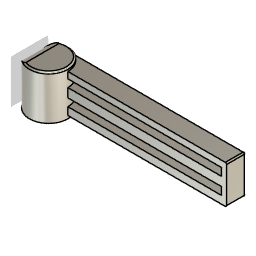
Link1 v24 (Autodesk Fusion 360 design; units mm, degrees)
Autodesk Fusion 360 part; units mm, degrees
sketch "Boceto1" plane through (0, 0, 0) normal (0, 1, 0) x (1, 0, 0)
  circle A0 centre (0, 0) radius 75.5
  dimension "d1" = 151
  constraint coincident A0.centre origin
  measures "d1" diameter of A0
extrude "Extruir1" add sketch "Boceto1" along normal blind 214.5
sketch "Boceto2" plane through (0, 0, 0) normal (1, 0, 0) x (0, 0, -1)
  line L0 (0, 201.5) -> (75, 201.5)
  line L1 (75, 201.5) -> (75, 51.5)
  line L2 (75, 51.5) -> (0, 51.5)
  line L3 (0, 51.5) -> (0, 201.5)
  line L4 (0, 176.5) -> (30, 176.5)
  line L5 (30, 176.5) -> (30, 146.5)
  line L6 (30, 146.5) -> (0, 146.5)
  line L7 (0, 146.5) -> (0, 176.5)
  line L8 (0, 111.5) -> (30, 111.5)
  line L9 (30, 111.5) -> (30, 81.5)
  line L10 (30, 81.5) -> (0, 81.5)
  line L11 (0, 81.5) -> (0, 111.5)
  point P0 (0, 214.5)
  dimension "d11" = 75
  dimension "d12" = 150
  dimension "d13" = 30
  dimension "d14" = 30
  dimension "d15" = 25
  dimension "d16" = 30
  dimension "d19" = 38
  dimension "d20" = 35
  constraint horizontal L0
  constraint vertical L1
  constraint horizontal L2
  constraint vertical L3
  constraint horizontal L4
  constraint vertical L5
  constraint horizontal L6
  constraint vertical L7
  constraint coincident L3 L4.start
  constraint horizontal L8
  constraint vertical L9
  constraint horizontal L10
  constraint vertical L11
  constraint coincident L3 L8.start
  measures "d11" distance of L0.start L0.end
  measures "d12" distance of L0.start L2.end
  measures "d13" distance of L4.start L4.end
  measures "d14" distance of L4.start L6.end
  measures "d15" distance of L0 L4
  measures "d16" distance of L2 L10
  measures "d19" distance of L4.start P0
  measures "d20" distance of L6 L8
sketch "Boceto3" plane through (0, 0, 0) normal (0, 0, 1) x (1, 0, 0)
sketch "Boceto4" plane through (0, 0, 0) normal (0, 0, 1) x (1, 0, 0)
  line L0 (-80, 0) -> (-80, 40)
  line L1 (-80, 40) -> (90, 40)
  line L2 (90, 40) -> (90, 0)
  line L3 (90, 0) -> (-80, 0)
  dimension "d8" = 40
  constraint vertical L0
  constraint perpendicular L0 L1
  constraint perpendicular L1 L2
  constraint perpendicular L0 L3
  measures "d8" distance of L0.start L0.end
extrude "Extruir3" cut sketch "Boceto4" along normal through all and the other way through all
extrude "Extruir4" add sketch "Boceto2" along normal blind 700 contours L0 L1 L2 L3 L4 L5 L6 L8 L9 L10
sketch "Boceto5" plane through (700, 0, 0) normal (1, 0, 0) x (0, 0, -1)
  line L0 (0, 111.5) -> (30, 111.5)
  line L1 (30, 111.5) -> (30, 81.5)
  line L2 (30, 81.5) -> (0, 81.5)
  line L3 (0, 81.5) -> (0, 51.5)
  line L4 (0, 51.5) -> (75, 51.5)
  line L5 (75, 51.5) -> (75, 201.5)
  line L6 (75, 201.5) -> (0, 201.5)
  line L7 (0, 201.5) -> (0, 176.5)
  line L8 (0, 176.5) -> (30, 176.5)
  line L9 (30, 176.5) -> (30, 146.5)
  line L10 (30, 146.5) -> (0, 146.5)
  line L11 (0, 146.5) -> (0, 111.5)
  line L12 (0, 176.5) -> (30, 176.5)
  line L13 (30, 176.5) -> (30, 146.5)
  line L14 (30, 146.5) -> (0, 146.5)
  line L15 (0, 146.5) -> (0, 176.5)
  line L16 (0, 111.5) -> (30, 111.5)
  line L17 (30, 111.5) -> (30, 81.5)
  line L18 (30, 81.5) -> (0, 81.5)
  line L19 (0, 81.5) -> (0, 111.5)
  constraint horizontal L12
  constraint vertical L13
  constraint horizontal L14
  constraint vertical L15
  constraint coincident L9.end L10.start
  constraint coincident L7.end L8.start
  constraint horizontal L16
  constraint vertical L17
  constraint horizontal L18
  constraint vertical L19
  constraint coincident L1.end L2.start
  constraint coincident L0.start L11.end
extrude "Extruir5" add sketch "Boceto5" against normal blind 20 contours L0 L1 L2 L16 L17 L18 L19 | L8 L9 L10 L12 L13 L14 L15
fillet "Empalme1" radius 6 1 edges at (-70.3907, 214.5, 27.302)
fillet "Empalme2" radius 5 1 edges at (700, 126.5, -75)
sketch "Boceto6" plane through (0, 0, 0) normal (0, 0, 1) x (1, 0, 0)
  spline S0 degree 5 poles (-140, 52.837) (-135.0375, 50.832) (-125.6476, 47.773) (-113.1693, 46.0387) (-99.7627, 49.465) (-88.3105, 63.072) (-81.5845, 84.6239) (-78.372, 111.348) (-76.0143, 137.2593) (-73.0835, 159.3989) (-68.896, 176.8089) (-63.175, 189.8686) (-55.7119, 199.6225) (-45.9985, 207.1017) (-32.9917, 212.8204) (-15.4222, 216.979) (3.2966, 219.0404) (20.4042, 219.8255) (33.2311, 220) (40, 220) knots 0 0 0 0 0 0 0.066667 0.133333 0.2 0.266667 0.333333 0.4 0.466667 0.533333 0.6 0.666667 0.733333 0.8 0.866667 0.933333 1 1 1 1 1 1
  line L0 (-0.2122, 220) -> (80.2122, 220)
  line L1 (-140, 52.837) -> (-140, 220)
  line L2 (-140, 220) -> (80.2122, 220)
  line L3 (-84.3539, 69.1429) -> (-75.6461, 130.8571)
  point P0 (-80, 100)
  point P1 (-56.9323, 197.1499)
  constraint midpoint S0.end L0
  constraint perpendicular L0 L1
  constraint coincident L0.end L2.end
  constraint perpendicular L1 L2
  constraint midpoint P0 L3
extrude "Extruir6" cut sketch "Boceto6" along normal through all and the other way through all
fillet "Fillet3" radius 5 6 edges at (351.8373, 201.5, -75) (698.5355, 201.5, -73.5355) (700, 201.5, -35) (351.8373, 51.5, -75) (698.5355, 51.5, -73.5355) (700, 51.5, -35)
sketch "Sketch7" plane through (0, 51.5, 0) normal (0, -1, 0) x (1, 0, 0)
  line L0 (695, -70) -> (695, 0)
move_body "Desplazar1" bodies 1 to x (1, 0, 0) y (0, 0, 1) z (0, -1, 0) at (0, 91.5, -161.5)
move_body "Desplazar2" bodies 1 to x (1, 0, 0) y (0, -1, 0) z (0, 0, -1) at (0, 213, 30)
move_body "Desplazar3" bodies 1 to x (1, 0, 0) y (0, 1, 0) z (0, 0, 1) at (-250, 0, -50)
move_body "Desplazar4" bodies 1 to x (-1, 0, 0) y (0, 1, 0) z (0, 0, -1) at (890, 0, -110)
move_body "Desplazar5" bodies 1 to x (0, -1, 0) y (1, 0, 0) z (0, 0, 1) at (393.5, 496.5, 0)
move_body "Desplazar6" bodies 1 to x (1, 0, 0) y (0, 1, 0) z (0, 0, 1) at (0, 650, 100)
move_body "Desplazar7" bodies 1 to x (1, 0, 0) y (0, 1, 0) z (0, 0, 1) at (-440, 0, -50)
move_body "Move8" bodies 1 to x (1, 0, 0) y (0, 1, 0) z (0, 0, 1) at (0, 0, 161.5)
move_body "Move9" bodies 1 to x (1, 0, 0) y (0, 1, 0) z (0, 0, 1) at (-75, -6.5, 0)
sketch "Sketch8" plane through (0, 0, 0) normal (0, 0, 1) x (1, 0, 0)
sketch "Sketch9" plane through (0, 0, 0) normal (1, 0, 0) x (0, 1, 0)
  line L0 (75.5, 0) -> (75.5, 71.5)
  line L1 (75.5, 71.5) -> (75.5, 106.5)
  dimension "d47" = 71.5
  dimension "d48" = 35
  constraint vertical L0
  constraint parallel L0 L1
  measures "d47" distance of L0.start L0.end
  measures "d48" distance of L0.end L1.end
sketch "Sketch10" plane through (0, 0, 0) normal (1, 0, 0) x (0, 1, 0)
  line L0 (75.5, 0) -> (75.5, 71.5)
  line L1 (680, 41.5) -> (75.5, 41.5)
  point P0 (700, 16.5)
  dimension "d49" = 700
  dimension "d50" = 75.5
  dimension "d51" = 604.5
  constraint coincident L0 L1.end
  constraint perpendicular L0 L1
  measures "d49" horizontal distance of origin P0
  measures "d50" distance of L0 origin
  measures "d51" distance of L1.start L1.end
